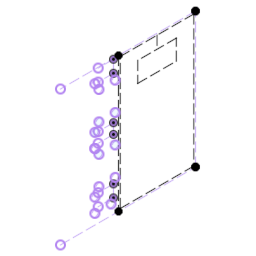
SAL v20 (Autodesk Fusion 360 design; units mm, degrees)
Autodesk Fusion 360 part; units mm, degrees
(part 1 of 3)
sketch "Sketch1" plane through (0, 0, 0) normal (0, 1, 0) x (1, 0, 0)
  line L0 (100, -100) -> (-100, -100) construction
  line L1 (-100, -100) -> (-100, 100) construction
  line L2 (-100, 100) -> (100, 100) construction
  line L3 (100, 100) -> (100, -100) construction
  line L4 (100, -100) -> (-100, 100) construction
  line L5 (-100, -100) -> (100, 100) construction
  line L6 (-105.5, -105.5) -> (-105.5, 105.5)
  line L7 (-105.5, 105.5) -> (105.5, 105.5)
  line L8 (105.5, 105.5) -> (105.5, -105.5)
  line L9 (105.5, -105.5) -> (-105.5, -105.5)
  line L10 (-95, -95) -> (-95, 95) construction
  line L11 (-95, 95) -> (95, 95) construction
  line L12 (95, 95) -> (95, -95) construction
  line L13 (95, -95) -> (-95, -95) construction
  line L14 (100, 100) -> (110, 100) construction
  line L15 (110, 100) -> (110, -100) construction
  line L16 (110, -100) -> (100, -100) construction
  line L17 (100, -100) -> (100, 100) construction
  line L18 (107.32, 100) -> (107.32, -100) construction
  line L19 (107.32, 90) -> (77.32, 90) construction
  line L20 (77.32, 90) -> (77.32, 10) construction
  line L21 (77.32, 10) -> (107.32, 10) construction
  line L22 (107.32, 10) -> (107.32, 90) construction
  line L23 (112.68, -100) -> (110, -100) construction
  line L24 (112.68, -100) -> (112.68, 100) construction
  line L25 (112.68, 100) -> (110, 100) construction
  line L26 (110, 0) -> (107.32, 0) construction
  line L27 (107.32, -100) -> (107.32, -105.5) construction
  line L28 (107.32, -105.5) -> (112.68, -105.5) construction
  line L29 (112.68, -105.5) -> (112.68, -100) construction
  line L30 (112.68, 100) -> (112.68, 105.5) construction
  line L31 (112.68, 105.5) -> (107.32, 105.5) construction
  line L32 (107.32, 105.5) -> (107.32, 100) construction
  line L33 (0, 0) -> (0, 110) construction
  line L34 (-100, 112.68) -> (100, 112.68)
  line L35 (100, 112.68) -> (100, 107.32)
  line L36 (100, 107.32) -> (-100, 107.32)
  line L37 (-100, 107.32) -> (-100, 112.68)
  line L38 (-100, 112.68) -> (100, 107.32) construction
  line L39 (100, 112.68) -> (-100, 107.32) construction
  line L40 (0, 0) -> (-105.5, 0) construction
  line L41 (100, -107.32) -> (-100, -107.32)
  line L42 (-88, -107.32) -> (-30, -107.32) construction
  line L43 (-30, -107.32) -> (-30, -42.32) construction
  line L44 (-30, -42.32) -> (-88, -42.32) construction
  line L45 (-88, -42.32) -> (-88, -107.32) construction
  line L46 (-107.32, 100) -> (-107.32, -100) construction
  line L47 (-112.68, -100) -> (-112.68, 100) construction
  point P0 (39.2, 88)
  point P1 (0, 110)
  dimension "d1" = 200
  dimension "d2" = -5.5
  dimension "d3" = 5
  dimension "d4" = 10
  dimension "d5" = 2.68
  dimension "d6" = 80
  dimension "d7" = 30
  dimension "d9" = 5
  dimension "d10" = 17.5
  dimension "d11" = 55.8
  dimension "d41" = 110
  dimension "d42" = 5.36
  dimension "d115" = 17.5
  dimension "d116" = 58
  dimension "d117" = 65
  constraint horizontal L0
  constraint perpendicular L0 L1
  constraint parallel L0 L2
  constraint parallel L1 L3
  constraint coincident L4 L33.start
  constraint coincident L5 L33.start
  constraint coincident L33.start L40.start
  constraint equal L2 L3
  constraint horizontal L14
  constraint vertical L15
  constraint horizontal L16
  constraint vertical L17
  constraint coincident L0.start L16
  constraint coincident L14 L18.start
  constraint coincident L16 L18.end
  constraint perpendicular L16 L18
  constraint horizontal L19
  constraint vertical L20
  constraint horizontal L21
  constraint vertical L22
  constraint coincident L18 L19.start
  constraint horizontal L23
  constraint perpendicular L23 L24
  constraint horizontal L25
  constraint midpoint L18 L26.end
  constraint midpoint L15 L26.start
  constraint equal L23 L26
  constraint perpendicular L16 L27
  constraint perpendicular L18 L28
  constraint coincident L23.start L24.start
  constraint vertical L29
  constraint coincident L8.end L28
  constraint perpendicular L25 L30
  constraint perpendicular L18 L31
  constraint perpendicular L14 L32
  constraint coincident L7.end L31
  constraint perpendicular L7 L33
  constraint horizontal L34
  constraint perpendicular L34 L35
  constraint parallel L34 L36
  constraint parallel L35 L37
  constraint coincident L38 P1
  constraint coincident L39 P1
  constraint coincident P1 L33.end
  constraint coincident L1.end L37
  constraint midpoint L6 L40.end
  constraint symmetric L35.end L40 L41.start
  constraint symmetric L36.end L40 L41.end
  constraint horizontal L42
  constraint vertical L43
  constraint horizontal L44
  constraint vertical L45
  constraint coincident L41 L42.start
  constraint symmetric L18.start L33 L46.start
  constraint symmetric L18.end L33 L46.end
  constraint symmetric L23.start L33 L47.start
  constraint symmetric L24.end L33 L47.end
  measures "d1" distance of L1.end L2.end
  measures "d4" distance of L15.end L0.start
  measures "d5" distance of L15 L18
  measures "d6" distance of L19.start L21.end
  measures "d7" distance of L20.end L21.end
  measures "d9" distance of L11.end L19
  measures "d10" distance of L7 P0
  measures "d11" distance of L12 P0
  measures "d41" distance of L33.start P1
  measures "d42" distance of L34.start L36.end
  measures "d115" distance of L6 L45
  measures "d116" distance of L42.start L42.end
  measures "d117" distance of L42.start L44.end
sketch "base_layer" plane through (0, 0, 0) normal (0, 1, 0) x (1, 0, 0)
  line L0 (-90, 90) -> (18, 90) construction
  line L1 (18, 90) -> (18, -10)
  line L2 (18, -10) -> (-90, -10) construction
  line L3 (-90, -10) -> (-90, 90) construction
  line L4 (-95, 95) -> (95, 95)
  line L5 (-68.2, 90) -> (-68.2, 39)
  line L6 (-68.2, 39) -> (-90, 39)
  line L7 (-87.5, -10) -> (-87.5, -6)
  line L8 (-82.5, -10) -> (-82.5, -6)
  arc A0 (-82.5, -6) -> (-87.5, -6) centre (-85, -6) ccw
  line L9 (-95, -95) -> (-95, 95)
  circle A1 centre (13, 87) radius 1.6
  circle A2 centre (-72.45, 43.25) radius 4.25
  line L10 (-90, 39) -> (-90, -10)
  line L11 (-87.5, -10) -> (-90, -10)
  line L12 (-82.5, -10) -> (18, -10)
  line L13 (-68.2, 90) -> (18, 90)
  circle A3 centre (22.25, 43.25) radius 4.25
  line L14 (-95, -95) -> (95, -95) construction
  line L15 (95, -95) -> (95, 95) construction
  line L16 (72.25, 90) -> (38.25, 90)
  line L17 (38.25, 90) -> (38.25, -6)
  line L18 (38.25, -6) -> (72.25, -6)
  line L19 (72.25, -6) -> (72.25, 90)
  line L20 (67.25, -6) -> (67.25, -1) construction
  line L21 (67.25, -1) -> (72.25, -1) construction
  line L22 (43.25, -6) -> (43.25, -1) construction
  line L23 (43.25, -1) -> (38.25, -1) construction
  line L24 (67.25, 90) -> (67.25, 85) construction
  line L25 (67.25, 85) -> (72.25, 85) construction
  line L26 (38.25, 85) -> (43.25, 85) construction
  line L27 (43.25, 85) -> (43.25, 90) construction
  line L28 (26.5, 43.25) -> (63.25, 43.25) construction
  line L29 (100, 100) -> (100, -100)
  line L30 (63.25, 90) -> (100, 90) construction
  point P0 (13, 87)
  point P1 (-63.2, 83.5)
  point P2 (-53.6, 83.5)
  point P3 (-44, 83.5)
  point P4 (-34.4, 83.5)
  point P5 (-24.8, 83.5)
  point P6 (5, 83.5)
  point P7 (63.25, 90)
  point P8 (67.25, -1)
  point P9 (43.25, -1)
  point P10 (43.25, 85)
  point P11 (67.25, 85)
  dimension "d12" = 100
  dimension "d13" = 108
  dimension "d14" = 5
  dimension "d15" = 51
  dimension "d16" = 21.8
  dimension "d17" = 3
  dimension "d18" = 5
  dimension "d19" = 2.5
  dimension "d20" = 5
  dimension "d21" = 4
  dimension "d22" = 5
  dimension "d23" = 3.2
  dimension "d28" = 9.6
  dimension "d29" = 0
  dimension "d30" = 5
  dimension "d31" = 13
  dimension "d38" = 8.5
  dimension "d39" = 6.5
  dimension "d52" = 5
  dimension "d54" = 34
  dimension "d55" = 96
  dimension "d56" = 9
  dimension "d57" = 5
  constraint horizontal L0
  constraint vertical L1
  constraint horizontal L2
  constraint vertical L3
  constraint coincident L0 L5.start
  constraint perpendicular L0 L5
  constraint coincident L3 L6.end
  constraint perpendicular L3 L6
  constraint coincident L2 L7.start
  constraint perpendicular L2 L7
  constraint coincident L2 L8.start
  constraint perpendicular L2 L8
  constraint horizontal L7.end L8.end
  constraint horizontal A0.centre L7.end
  constraint coincident L7.end A0.end
  constraint coincident P0 A1.centre
  constraint horizontal P5 P6
  constraint tangent L5 A2
  constraint tangent L6 A2
  constraint coincident L5.start L13.start
  constraint equal A2 A3
  constraint horizontal A2.centre A3.centre
  constraint tangent L1 A3
  constraint coincident L9.start L14.start
  constraint perpendicular L9 L14
  constraint coincident L4.end L15.end
  constraint vertical L15
  constraint horizontal L16
  constraint vertical L17
  constraint horizontal L18
  constraint vertical L19
  constraint coincident L16 P7
  constraint coincident L18 L20.start
  constraint perpendicular L18 L20
  constraint coincident L19 L21.end
  constraint perpendicular L19 L21
  constraint coincident L18 L22.start
  constraint perpendicular L18 L22
  constraint coincident L17 L23.end
  constraint perpendicular L17 L23
  constraint coincident L19 L25.end
  constraint perpendicular L19 L25
  constraint coincident L17 L26.start
  constraint perpendicular L17 L26
  constraint vertical L27
  constraint equal L26 L27
  constraint equal L24 L27
  constraint equal L24 L25
  constraint equal L23 L26
  constraint equal L22 L23
  constraint equal L20 L22
  constraint equal L20 L21
  constraint coincident P8 L20.end
  constraint coincident P9 L22.end
  constraint coincident P10 L26.end
  constraint coincident P11 L24.end
  constraint coincident A3 L28.start
  constraint perpendicular L17 L28
  constraint coincident A3.centre L28
  constraint vertical P7 L28.end
  constraint coincident L16 L27.end
  constraint coincident P7 L30.start
  constraint coincident L29 L30.end
  constraint perpendicular L29 L30
  constraint equal L28 L30
  constraint coincident L16 L24.start
  constraint vertical L24
  measures "d12" distance of L0.end L1.end
  measures "d13" distance of L0.start L0.end
  measures "d14" distance of L0 L4
  measures "d15" distance of L0 L6
  measures "d16" distance of L3 L5
  measures "d17" vertical distance of L0.end P0
  measures "d18" horizontal distance of L0.end P0
  measures "d19" distance of L2.end L7
  measures "d20" distance of L7 L8
  measures "d21" distance of L2 A0.centre
  measures "d22" distance of L3 L9
  measures "d23" diameter of A1
  measures "d30" distance of L5 P1
  measures "d31" distance of L1 P6
  measures "d38" diameter of A2
  measures "d39" distance of L0 P6
  measures "d52" distance of L4 L16
  measures "d54" distance of L16.start L16.end
  measures "d55" distance of L16.start L18.end
  measures "d56" distance of L16.start P7
  measures "d57" distance of L26.start P10
sketch "switch_screw_plan" plane through (0, 0, 0) normal (1, 0, 0) x (0, 0, -1)
  line L0 (0, 0) -> (0, 2.68) construction
  line L1 (0, 0) -> (0, -2.68) construction
  line L2 (0, 0) -> (10, 0) construction
  line L3 (10, 0) -> (10, 20) construction
  line L4 (10, 20) -> (0, 20) construction
  line L5 (0, 20) -> (0, 12) construction
  line L6 (0, 12) -> (0, 2.68)
  point P0 (0, 12)
  point P1 (0, 2.68)
  point P2 (0, 13.6)
  dimension "d32" = 5.36
  dimension "d33" = 10
  dimension "d34" = 20
  dimension "d35" = 8
  dimension "d36" = 9.32
  dimension "d37" = 1.6
  constraint coincident L0.start L1.start
  constraint vertical L0
  constraint parallel L0 L1
  constraint equal L0 L1
  constraint perpendicular L0 L2
  constraint perpendicular L2 L3
  constraint perpendicular L3 L4
  constraint coincident L0 L4.end
  constraint perpendicular L4 L5
  constraint coincident P0 L5.end
  constraint coincident P1 L0.end
  constraint coincident L5 P2
  measures "d32" distance of P1 L1.end
  measures "d33" distance of L0.start L2.end
  measures "d34" distance of L2.end L3.end
  measures "d35" distance of L4.end P0
  measures "d36" distance of P1 P0
  measures "d37" distance of P0 P2
sketch "back_board_0" plane through (0, 0, 0) normal (0, 0, 1) x (1, 0, 0)
  line L0 (0, 0) -> (0, 10) construction
  line L1 (0, 0) -> (0, -10) construction
  line L2 (0, 10) -> (0, 30) construction
  line L3 (0, 30) -> (0, 35.5) construction
  line L4 (100, 35.5) -> (-100, 35.5)
  line L5 (-100, 35.5) -> (-100, 4.5) construction
  line L6 (-100, 4.5) -> (100, 4.5)
  line L7 (100, 4.5) -> (100, 35.5) construction
  line L8 (100, 35.5) -> (-100, 4.5) construction
  line L9 (-100, 35.5) -> (100, 4.5) construction
  circle A0 centre (5, 20) radius 2.25
  circle A1 centre (-24.8, 20) radius 2.25
  circle A2 centre (-34.4, 20) radius 2.25
  circle A3 centre (-63.2, 20) radius 2.25
  circle A4 centre (-53.6, 20) radius 2.25
  circle A5 centre (-44, 20) radius 2.25
  line L10 (26.5, 0) -> (18, 0)
  line L11 (29.5, 4.5) -> (29.5, 35.5) construction
  line L12 (29.5, 20) -> (100, 20) construction
  line L13 (52.25, 20) -> (77.25, 20) construction
  circle A6 centre (52.25, 20) radius 1.1
  circle A7 centre (77.25, 20) radius 1.1
  line L14 (55.35, 14.2) -> (74.15, 14.2) construction
  line L15 (74.15, 14.2) -> (74.15, 25.8) construction
  line L16 (74.15, 25.8) -> (55.35, 25.8) construction
  line L17 (55.35, 25.8) -> (55.35, 14.2)
  line L18 (55.35, 14.2) -> (74.15, 25.8) construction
  line L19 (74.15, 14.2) -> (55.35, 25.8) construction
  arc A8 (74.15, 21.8) -> (70.15, 25.8) centre (70.15, 21.8) ccw
  arc A9 (70.15, 14.2) -> (74.15, 18.2) centre (70.15, 18.2) ccw
  line L20 (74.15, 18.2) -> (74.15, 21.8)
  line L21 (70.15, 25.8) -> (55.35, 25.8)
  line L22 (70.15, 14.2) -> (55.35, 14.2)
  line L23 (105.5, 0) -> (-105.5, 0)
  line L24 (-100, 4.5) -> (-105.5, 4.5)
  line L25 (-105.5, 4.5) -> (-105.5, 35.5)
  line L26 (-105.5, 35.5) -> (-100, 35.5)
  line L27 (100, 4.5) -> (105.5, 4.5)
  line L28 (105.5, 4.5) -> (105.5, 35.5)
  line L29 (105.5, 35.5) -> (100, 35.5)
  point P0 (0, 4.5)
  point P1 (0, 20)
  point P2 (100, 0)
  point P3 (0, 20)
  point P4 (5, 0)
  point P5 (-24.8, 0)
  point P6 (-34.4, 0)
  point P7 (-44, 0)
  point P8 (-53.6, 0)
  point P9 (-63.2, 0)
  point P10 (5, 20)
  point P11 (-24.8, 20)
  point P12 (-34.4, 20)
  point P13 (-44, 20)
  point P14 (-53.6, 20)
  point P15 (-63.2, 20)
  point P16 (64.75, 20)
  point P17 (52.25, 20)
  point P18 (77.25, 20)
  point P19 (64.75, 20)
  dimension "d43" = 20
  dimension "d44" = 20
  dimension "d45" = 5.5
  dimension "d46" = 5.5
  dimension "d47" = 4.5
  dimension "d51" = 3
  dimension "d104" = 25
  dimension "d105" = 2.2
  dimension "d106" = 18.8
  dimension "d107" = 11.6
  dimension "d108" = 4
  constraint coincident L0.start L1.start
  constraint vertical L0
  constraint parallel L0 L1
  constraint equal L0 L1
  constraint parallel L0 L2
  constraint coincident L0 P0
  constraint parallel L2 L3
  constraint midpoint L2 P3
  constraint horizontal L4
  constraint perpendicular L4 L5
  constraint parallel L4 L6
  constraint parallel L5 L7
  constraint coincident L8 P3
  constraint coincident L9 P3
  constraint coincident P3 P1
  constraint coincident P2 L7
  constraint coincident P0 L6
  constraint vertical P9 P15
  constraint vertical P8 P14
  constraint vertical P7 P13
  constraint vertical P6 P12
  constraint vertical P5 P11
  constraint vertical P4 P10
  constraint horizontal P3 P10
  constraint horizontal P3 P11
  constraint horizontal P3 P12
  constraint horizontal P3 P13
  constraint horizontal P3 P14
  constraint horizontal P3 P15
  constraint coincident P10 A0.centre
  constraint coincident P11 A1.centre
  constraint coincident P12 A2.centre
  constraint coincident P15 A3.centre
  constraint coincident P14 A4.centre
  constraint coincident P13 A5.centre
  constraint equal A0 A1
  constraint equal A1 A2
  constraint equal A1 A5
  constraint equal A1 A4
  constraint equal A1 A3
  constraint coincident L6 L11.start
  constraint coincident L4 L11.end
  constraint perpendicular L4 L11
  constraint midpoint L11 L12.start
  constraint midpoint L7 L12.end
  constraint midpoint L12 P19
  constraint coincident L12 P17
  constraint coincident L12 P18
  constraint coincident P17 L13.start
  constraint coincident P18 L13.end
  constraint parallel L12 L13
  constraint midpoint P19 L13
  constraint equal A6 A7
  constraint horizontal L14
  constraint perpendicular L14 L15
  constraint parallel L14 L16
  constraint parallel L15 L17
  constraint coincident L18 P19
  constraint coincident L19 P19
  constraint coincident P19 P16
  constraint horizontal A8.centre A8.start
  constraint vertical A8.centre A8.end
  constraint coincident L16 A8.end
  constraint coincident L15 A8.start
  constraint horizontal A9.centre A9.end
  constraint vertical A9.centre A9.start
  constraint equal A8 A9
  constraint coincident L15 A9.end
  constraint coincident L14 A9.start
  constraint coincident A9.end L20.start
  constraint perpendicular L5 L24
  constraint perpendicular L24 L25
  constraint horizontal L26
  constraint coincident L23.end L25
  constraint perpendicular L7 L27
  constraint perpendicular L27 L28
  constraint horizontal L29
  constraint coincident L23.start L28
  measures "d43" distance of L0.end L1.end
  measures "d44" distance of L0.end L2.end
  measures "d45" distance of L2.end L3.end
  measures "d46" distance of L0.end P0
  measures "d47" diameter of A0
  measures "d51" horizontal distance of L10.start L11.start
  measures "d104" distance of P17 P18
  measures "d105" diameter of A6
  measures "d106" distance of L15.end L16.end
  measures "d107" distance of L14.end L15.end
  measures "d108" radius of A8
sketch "left side panel" plane through (0, 0, 0) normal (1, 0, 0) x (0, 0, -1)
  line L0 (-120, 10) -> (120, 10) construction
  line L1 (120, 10) -> (120, -10) construction
  line L2 (120, -10) -> (-120, -10) construction
  line L3 (-120, -10) -> (-120, 10) construction
  line L4 (-120, 10) -> (120, -10) construction
  line L5 (120, 10) -> (-120, -10) construction
  line L6 (120, 10) -> (120, 230) construction
  line L7 (120, 230) -> (-120, 230) construction
  line L8 (-120, 230) -> (-120, 10) construction
  line L9 (-105.5, 215.5) -> (105.5, 215.5)
  line L10 (105.5, 215.5) -> (105.5, 4.5)
  line L11 (105.5, 4.5) -> (-105.5, 4.5)
  line L12 (-105.5, 4.5) -> (-105.5, 215.5)
  line L13 (-105.5, 215.5) -> (-120, 215.5) construction
  line L14 (-120, 215.5) -> (-120, 230) construction
  line L15 (-120, 230) -> (-105.5, 230) construction
  line L16 (-105.5, 230) -> (-105.5, 215.5) construction
  line L17 (-100, 10) -> (100, 10) construction
  line L18 (100, 10) -> (100, 210) construction
  line L19 (100, 210) -> (-100, 210) construction
  line L20 (-100, 210) -> (-100, 10) construction
  line L21 (100, 210) -> (105.5, 210) construction
  line L22 (105.5, 210) -> (105.5, 215.5) construction
  line L23 (105.5, 215.5) -> (100, 215.5) construction
  line L24 (100, 215.5) -> (100, 210) construction
  line L25 (10, 95) -> (90, 95) construction
  line L26 (90, 95) -> (90, 15) construction
  line L27 (90, 15) -> (10, 15) construction
  line L28 (10, 15) -> (10, 95) construction
  line L29 (10, 192.5) -> (90, 192.5) construction
  line L30 (90, 192.5) -> (90, 112.5) construction
  line L31 (90, 112.5) -> (10, 112.5) construction
  line L32 (10, 112.5) -> (10, 192.5) construction
  line L33 (90, 192.5) -> (90, 210) construction
  line L34 (90, 95) -> (90, 112.5) construction
  line L35 (10, 95) -> (14.25, 95) construction
  line L36 (14.25, 95) -> (14.25, 90.75) construction
  line L37 (14.25, 90.75) -> (10, 90.75) construction
  line L38 (10, 90.75) -> (10, 95) construction
  line L39 (90, 95) -> (85.75, 95) construction
  line L40 (85.75, 95) -> (85.75, 90.75) construction
  line L41 (85.75, 90.75) -> (90, 90.75) construction
  line L42 (90, 90.75) -> (90, 95) construction
  line L43 (10, 15) -> (14.25, 15) construction
  line L44 (14.25, 15) -> (14.25, 19.25) construction
  line L45 (14.25, 19.25) -> (10, 19.25) construction
  line L46 (10, 19.25) -> (10, 15) construction
  line L47 (90, 15) -> (85.75, 15) construction
  line L48 (85.75, 15) -> (85.75, 19.25) construction
  line L49 (85.75, 19.25) -> (90, 19.25) construction
  line L50 (90, 19.25) -> (90, 15) construction
  line L51 (90, 112.5) -> (85.75, 112.5) construction
  line L52 (85.75, 112.5) -> (85.75, 116.75) construction
  line L53 (85.75, 116.75) -> (90, 116.75) construction
  line L54 (90, 116.75) -> (90, 112.5) construction
  line L55 (90, 192.5) -> (85.75, 192.5) construction
  line L56 (85.75, 192.5) -> (85.75, 188.25) construction
  line L57 (85.75, 188.25) -> (90, 188.25) construction
  line L58 (90, 188.25) -> (90, 192.5) construction
  line L59 (10, 192.5) -> (14.25, 192.5) construction
  line L60 (14.25, 192.5) -> (14.25, 188.25) construction
  line L61 (14.25, 188.25) -> (10, 188.25) construction
  line L62 (10, 188.25) -> (10, 192.5) construction
  line L63 (10, 112.5) -> (14.25, 112.5) construction
  line L64 (14.25, 112.5) -> (14.25, 116.75) construction
  line L65 (14.25, 116.75) -> (10, 116.75) construction
  line L66 (10, 116.75) -> (10, 112.5) construction
  line L67 (90, 15) -> (90, 10) construction
  line L68 (14.25, 19.25) -> (85.75, 90.75) construction
  circle A0 centre (50, 55) radius 43.5 construction
  circle A1 centre (14.25, 90.75) radius 2.5
  circle A2 centre (85.75, 90.75) radius 2.5
  circle A3 centre (14.25, 19.25) radius 2.5
  circle A4 centre (85.75, 19.25) radius 2.5
  arc A5 (32.9047, 95) -> (10, 72.0953) centre (50, 55) ccw
  arc A6 (90, 72.0953) -> (67.0953, 95) centre (50, 55) ccw
  arc A7 (67.0953, 15) -> (90, 37.9047) centre (50, 55) ccw
  arc A8 (10, 37.9047) -> (32.9047, 15) centre (50, 55) ccw
  line L69 (10, 72.0953) -> (10, 37.9047)
  line L70 (32.9047, 15) -> (67.0953, 15)
  line L71 (90, 37.9047) -> (90, 72.0953)
  line L72 (67.0953, 95) -> (32.9047, 95)
  line L73 (90, 103.75) -> (10, 103.75) construction
  circle A9 centre (85.75, 116.75) radius 2.5
  circle A10 centre (14.25, 116.75) radius 2.5
  arc A11 (10, 135.4047) -> (32.9047, 112.5) centre (50, 152.5) ccw
  line L74 (67.0953, 112.5) -> (32.9047, 112.5)
  arc A12 (90, 169.5953) -> (67.0953, 192.5) centre (50, 152.5) ccw
  line L75 (32.9047, 192.5) -> (67.0953, 192.5)
  arc A13 (32.9047, 192.5) -> (10, 169.5953) centre (50, 152.5) ccw
  line L76 (10, 135.4047) -> (10, 169.5953)
  arc A14 (67.0953, 112.5) -> (90, 135.4047) centre (50, 152.5) ccw
  line L77 (90, 169.5953) -> (90, 135.4047)
  circle A15 centre (85.75, 188.25) radius 2.5
  circle A16 centre (14.25, 188.25) radius 2.5
  point P0 (0, 4.5)
  point P1 (0, 10)
  point P2 (90, 0)
  point P3 (85.75, 188.25)
  point P4 (14.25, 188.25)
  point P5 (14.25, 116.75)
  point P6 (85.75, 116.75)
  point P7 (85.75, 90.75)
  point P8 (14.25, 19.25)
  point P9 (14.25, 90.75)
  point P10 (85.75, 19.25)
  point P11 (90, 0)
  point P12 (50, 55)
  point P13 (-0.7942, 92.6847)
  dimension "d58" = 240
  dimension "d59" = 20
  dimension "d60" = 240
  dimension "d61" = 5.5
  dimension "d62" = 80
  dimension "d64" = 4.25
  dimension "d65" = 5
  dimension "d66" = 87
  dimension "d82" = 5
  constraint horizontal L0
  constraint perpendicular L0 L1
  constraint parallel L0 L2
  constraint parallel L1 L3
  constraint coincident L4 origin
  constraint coincident L5 origin
  constraint vertical L6
  constraint horizontal L7
  constraint vertical L8
  constraint coincident L0.end L1.start
  constraint horizontal L9
  constraint vertical L10
  constraint horizontal L11
  constraint vertical L12
  constraint midpoint L11 P0
  constraint vertical origin P0
  constraint equal L9 L10
  constraint horizontal L13
  constraint vertical L14
  constraint horizontal L15
  constraint vertical L16
  constraint equal L13 L16
  constraint horizontal L17
  constraint vertical L18
  constraint horizontal L19
  constraint vertical L20
  constraint coincident L0 L17.start
  constraint midpoint L17 P1
  constraint vertical P0 P1
  constraint equal L18 L19
  constraint horizontal L21
  constraint vertical L22
  constraint horizontal L23
  constraint vertical L24
  constraint equal L21 L24
  constraint horizontal L25
  constraint vertical L26
  constraint horizontal L27
  constraint vertical L28
  constraint equal L25 L28
  constraint horizontal L29
  constraint vertical L30
  constraint horizontal L31
  constraint vertical L32
  constraint equal L29 L30
  constraint collinear L26 L30
  constraint coincident L19 L33.end
  constraint perpendicular L19 L33
  constraint perpendicular L31 L34
  constraint equal L33 L34
  constraint horizontal L35
  constraint vertical L36
  constraint horizontal L37
  constraint vertical L38
  constraint horizontal L39
  constraint vertical L40
  constraint horizontal L41
  constraint vertical L42
  constraint horizontal L43
  constraint vertical L44
  constraint horizontal L45
  constraint vertical L46
  constraint horizontal L47
  constraint vertical L48
  constraint horizontal L49
  constraint vertical L50
  constraint horizontal L51
  constraint vertical L52
  constraint horizontal L53
  constraint vertical L54
  constraint horizontal L55
  constraint vertical L56
  constraint horizontal L57
  constraint vertical L58
  constraint horizontal L59
  constraint vertical L60
  constraint horizontal L61
  constraint vertical L62
  constraint horizontal L63
  constraint vertical L64
  constraint horizontal L65
  constraint vertical L66
  constraint equal L36 L37
  constraint equal L36 L64
  constraint equal L64 L65
  constraint equal L36 L40
  constraint equal L40 L41
  constraint equal L41 L49
  constraint equal L48 L49
  constraint equal L37 L45
  constraint equal L44 L45
  constraint equal L52 L64
  constraint equal L52 L53
  constraint equal L53 L57
  constraint equal L56 L57
  constraint equal L61 L65
  constraint equal L60 L61
  constraint coincident P3 L56.end
  constraint coincident P4 L60.end
  constraint coincident P5 L64.end
  constraint coincident P6 L52.end
  constraint coincident P7 L40.end
  constraint coincident P8 L44.end
  constraint coincident P9 L36.end
  constraint coincident P10 L48.end
  constraint coincident L0 L67.end
  constraint vertical L67
  constraint coincident L67 P11
  constraint midpoint L68 P12
  constraint coincident P12 A0.centre
  constraint equal A1 A2
  constraint equal A3 A4
  constraint equal A1 A3
  constraint coincident A0 A5.end
  constraint coincident L28 A5.end
  constraint coincident A0 A6.end
  constraint coincident L25 A6.end
  constraint coincident A0 A7.end
  constraint coincident L26 A7.end
  constraint coincident L28 A8.start
  constraint coincident L27 A8.end
  constraint coincident A0 A8.end
  constraint perpendicular L70 L71
  constraint perpendicular L71 L72
  constraint horizontal L70
  constraint midpoint L34 L73.start
  constraint perpendicular L34 L73
  constraint coincident L32 L73.end
  constraint symmetric A1 L73 A10
  constraint symmetric A2 L73 A9
  constraint symmetric A3 L73 A16
  constraint symmetric A4 L73 A15
  constraint symmetric A5.start L73 A11.end
  constraint symmetric A5.end L73 A11.start
  constraint symmetric A5 L73 A11
  constraint symmetric A6.start L73 A14.end
  constraint symmetric A6.end L73 L74.start
  constraint symmetric A6 L73 A14
  constraint symmetric A7.start L73 A12.end
  constraint symmetric A7.end L73 A12.start
  constraint symmetric A7 L73 A12
  constraint symmetric A8.start L73 A13.end
  constraint symmetric A8.end L73 L75.start
  constraint symmetric A8 L73 A13
  constraint equal L25 L29
  measures "d58" distance of L1.end L2.end
  measures "d59" distance of L0.end L1.end
  measures "d60" distance of L2.end L7.end
  measures "d61" distance of L0 L11
  measures "d62" distance of L25.start L25.end
  measures "d64" distance of P9 L37.end
  measures "d65" distance of L26.end L67.end
  measures "d66" diameter of A0
  measures "d82" diameter of A1
sketch "vertical_planning" plane through (0, 0, 0) normal (0, 0, 1) x (1, 0, 0)
  line L0 (100, 10) -> (-100, 10)
  line L1 (-100, 10) -> (-100, -10)
  line L2 (-100, -10) -> (100, -10)
  line L3 (100, -10) -> (100, 10)
  line L4 (100, 10) -> (-100, -10) construction
  line L5 (-100, 10) -> (100, -10) construction
  line L6 (100, 30) -> (-100, 30)
  line L7 (-100, 30) -> (-100, 10)
  line L8 (100, 10) -> (100, 30)
  line L9 (100, 50) -> (-100, 50)
  line L10 (-100, 50) -> (-100, 30)
  line L11 (100, 30) -> (100, 50)
  line L12 (100, 70) -> (-100, 70)
  line L13 (-100, 70) -> (-100, 50)
  line L14 (100, 50) -> (100, 70)
  line L15 (100, 90) -> (-100, 90)
  line L16 (-100, 90) -> (-100, 70)
  line L17 (100, 70) -> (100, 90)
  line L18 (100, 110) -> (-100, 110)
  line L19 (-100, 110) -> (-100, 90)
  line L20 (100, 90) -> (100, 110)
  line L21 (100, 130) -> (-100, 130)
  line L22 (-100, 130) -> (-100, 110)
  line L23 (100, 110) -> (100, 130)
  line L24 (100, 150) -> (-100, 150)
  line L25 (-100, 150) -> (-100, 130)
  line L26 (100, 130) -> (100, 150)
  line L27 (100, 170) -> (-100, 170)
  line L28 (-100, 170) -> (-100, 150)
  line L29 (100, 150) -> (100, 170)
  line L30 (100, 190) -> (-100, 190)
  line L31 (-100, 190) -> (-100, 170)
  line L32 (100, 170) -> (100, 190)
  line L33 (100, 210) -> (-100, 210)
  line L34 (-100, 210) -> (-100, 190)
  line L35 (100, 190) -> (100, 210)
  line L36 (100, 230) -> (-100, 230)
  line L37 (-100, 230) -> (-100, 210)
  line L38 (100, 210) -> (100, 230)
  line L39 (-100, 40) -> (100, 40) construction
  line L40 (-100, 80) -> (100, 80) construction
  line L41 (100, 120) -> (-100, 120) construction
  line L42 (-100, 160) -> (100, 160) construction
  line L43 (100, 200) -> (-100, 200) construction
  line L44 (100, 42.675) -> (-100, 42.675)
  line L45 (100, 37.325) -> (-100, 37.325)
  line L46 (-100, 82.675) -> (100, 82.675)
  line L47 (-100, 77.325) -> (100, 77.325)
  line L48 (100, 122.675) -> (-100, 122.675)
  line L49 (100, 162.675) -> (-100, 162.675)
  line L50 (100, 202.675) -> (-100, 202.675)
  line L51 (100, 197.325) -> (-100, 197.325)
  line L52 (100, 157.325) -> (-100, 157.325)
  line L53 (100, 117.325) -> (-100, 117.325)
  point P0 (-100, 0)
  point P1 (0, 10)
  dimension "d86" = 0
  dimension "d87" = 220
  dimension "d308" = 2.675
  dimension "d309" = 2.675
  dimension "d310" = 2.675
  dimension "d311" = 2.675
  dimension "d312" = 2.675
  constraint horizontal L0
  constraint perpendicular L0 L1
  constraint parallel L0 L2
  constraint parallel L1 L3
  constraint coincident L4 origin
  constraint coincident L5 origin
  constraint coincident P1 L0
  constraint coincident P0 L1
  constraint midpoint L10 L39.start
  constraint midpoint L11 L39.end
  constraint midpoint L16 L40.start
  constraint midpoint L17 L40.end
  constraint midpoint L23 L41.start
  constraint midpoint L22 L41.end
  constraint midpoint L28 L42.start
  constraint midpoint L29 L42.end
  constraint midpoint L35 L43.start
  constraint midpoint L34 L43.end
  constraint coincident L11 L44.start
  constraint coincident L10 L44.end
  constraint perpendicular L10 L44
  constraint symmetric L39 L44.start L45.start
  constraint symmetric L39 L44.end L45.end
  constraint coincident L16 L46.start
  constraint coincident L17 L46.end
  constraint perpendicular L17 L46
  constraint symmetric L40 L46.start L47.start
  constraint symmetric L40 L46.end L47.end
  constraint coincident L23 L48.start
  constraint coincident L22 L48.end
  constraint perpendicular L22 L48
  constraint coincident L29 L49.start
  constraint coincident L28 L49.end
  constraint perpendicular L28 L49
  constraint coincident L35 L50.start
  constraint coincident L34 L50.end
  constraint perpendicular L34 L50
  constraint symmetric L43 L50.start L51.start
  constraint symmetric L43 L50.end L51.end
  constraint symmetric L42 L49.start L52.start
  constraint symmetric L42 L49.end L52.end
  constraint symmetric L41 L48.start L53.start
  constraint symmetric L41 L48.end L53.end
  measures "d308" distance of L39 L44
  measures "d309" distance of L40 L46
  measures "d310" distance of L41 L48
  measures "d311" distance of L42 L49
  measures "d312" distance of L43 L50
extrude "Extrude1" add sketch "base_layer" along normal up to surface (1.6 mm away) from surface at 12 contours L1 L5 L6 L7 L8 A0 L10 L11 L12 L13 makes body 1
sketch "standoffs" plane through (0, 0, 0) normal (0, 1, 0) x (1, 0, 0)
  circle A0 centre (-72.45, 43.25) radius 4.25
  circle A1 centre (22.25, 43.25) radius 4.25
  circle A2 centre (-72.45, 43.25) radius 2.7
  circle A3 centre (-85, -6) radius 4.25
  circle A4 centre (22.25, 43.25) radius 2.7
  circle A5 centre (13, 87) radius 1.75
  circle A6 centre (13, 87) radius 4.25
  circle A7 centre (-85, -6) radius 2.7
  point P0 (-85, -6)
  point P1 (13, 87)
  dimension "d91" = 5.4
  dimension "d92" = 3.5
  constraint concentric A0 A2
  constraint coincident P0 A3.centre
  constraint concentric A1 A4
  constraint coincident P1 A5.centre
  constraint concentric A5 A6
  constraint equal A0 A3
  constraint equal A2 A4
  constraint equal A1 A6
  constraint equal A2 A7
  measures "d91" diameter of A2
  measures "d92" diameter of A5
extrude "Extrude2" add sketch "standoffs" along normal up to surface (9.12 mm away) from surface at 2.68 separate body contours A3 | A6 makes body 2 at (17.2447, 8.76, -86.7882) makes body 3 at (-80.7553, 8.76, 6.2118)
extrude "Extrude3" add sketch "standoffs" along normal blind 7 from surface at 2.68 separate body contours A0 | A1 makes body 4 at (26.4789, 7.3467, -42.8268) makes body 5 at (-68.2211, 7.3467, -42.8268)
sketch "bottom board laser cut" plane through (0, 0, 0) normal (0, 1, 0) x (1, 0, 0)
  line L0 (-105.5, -105.5) -> (-105.5, 105.5)
  line L1 (-105.5, 105.5) -> (105.5, 105.5)
  line L2 (105.5, 105.5) -> (105.5, -105.5)
  line L3 (105.5, -105.5) -> (-105.5, -105.5)
  line L4 (-90, -10) -> (-90, 90) construction
  line L5 (-90, 90) -> (18, 90) construction
  line L6 (95, -95) -> (95, 95) construction
  line L7 (-95, -95) -> (95, -95) construction
  circle A0 centre (-85, -6) radius 2
  circle A1 centre (-72.45, 43.25) radius 2
  circle A2 centre (22.25, 43.25) radius 2
  circle A3 centre (13, 87) radius 1.1
  circle A4 centre (43.25, -1) radius 0.9
  circle A5 centre (67.25, -1) radius 0.9
  circle A6 centre (67.25, 85) radius 0.9
  circle A7 centre (43.25, 85) radius 0.9
  line L8 (95, -95) -> (5, -95) construction
  line L9 (5, -95) -> (5, -80) construction
  line L10 (5, -80) -> (95, -80) construction
  line L11 (95, -80) -> (95, -95) construction
  circle A8 centre (5, -80) radius 0.9
  point P0 (-72.45, 43.25)
  point P1 (-85, -6)
  point P2 (22.25, 43.25)
  point P3 (13, 87)
  point P4 (43.25, -1)
  point P5 (67.25, -1)
  point P6 (67.25, 85)
  point P7 (43.25, 85)
  dimension "d99" = 4
  dimension "d100" = 2.2
  dimension "d101" = 1.8
  dimension "d102" = 90
  dimension "d103" = 15
  constraint coincident P1 A0.centre
  constraint coincident P0 A1.centre
  constraint coincident P2 A2.centre
  constraint coincident P3 A3.centre
  constraint coincident P4 A4.centre
  constraint coincident P5 A5.centre
  constraint coincident P6 A6.centre
  constraint coincident P7 A7.centre
  constraint equal A4 A5
  constraint equal A4 A7
  constraint equal A4 A6
  constraint equal A0 A1
  constraint equal A0 A2
  constraint horizontal L8
  constraint vertical L9
  constraint horizontal L10
  constraint vertical L11
  constraint coincident L6.start L7.end
  constraint coincident L9.end L10.start
  constraint equal A4 A8
  measures "d99" diameter of A0
  measures "d100" diameter of A3
  measures "d101" diameter of A4
  measures "d102" distance of L6.start L8.end
  measures "d103" distance of L6.start L10.end
sketch "amplifier_support" plane through (0, 0, 0) normal (0, 1, 0) x (1, 0, 0)
  line L0 (-2.5, -76.5) -> (12.5, -76.5) construction
  line L1 (12.5, -76.5) -> (12.5, -83.5)
  line L2 (12.5, -83.5) -> (-2.5, -83.5)
  line L3 (-2.5, -83.5) -> (-2.5, -76.5)
  line L4 (-2.5, -76.5) -> (12.5, -83.5) construction
  line L5 (12.5, -76.5) -> (-2.5, -83.5) construction
  line L6 (12.5, -76.5) -> (12.5, -74.5)
  line L7 (12.5, -74.5) -> (-2.5, -74.5)
  line L8 (-2.5, -74.5) -> (-2.5, -76.5)
  circle A0 centre (5, -80) radius 1.3
  point P0 (5, -80)
  point P1 (5, -80)
  dimension "d109" = 15
  dimension "d110" = 7
  dimension "d111" = 2
  dimension "d112" = 2.6
  constraint horizontal L0
  constraint perpendicular L0 L1
  constraint parallel L0 L2
  constraint parallel L1 L3
  constraint coincident L4 P1
  constraint coincident L5 P1
  constraint coincident P0 A0.centre
  constraint perpendicular L0 L6
  constraint perpendicular L6 L7
  constraint vertical L8
  constraint coincident P1 P0
  measures "d109" distance of L1.end L2.end
  measures "d110" distance of L0.end L1.end
  measures "d111" distance of L0.start L7.end
  measures "d112" diameter of A0
extrude "Extrude4" add sketch "amplifier_support" along normal blind 3 separate body makes body 6
sketch "Sketch10" plane through (0, 0, 0) normal (0, 0, 1) x (1, 0, 0)
  point P0 (100, 40)
  point P1 (100, 80)
  point P2 (100, 120)
  point P3 (100, 160)
  point P4 (100, 200)
  point P5 (77.32, 0)
sketch "intraboard_planning" plane through (0, 0, 0) normal (0, 1, 0) x (1, 0, 0)
  line L0 (-105.5, 105.5) -> (105.5, 105.5)
  line L1 (-30, -42.32) -> (-88, -42.32)
  line L2 (77.32, 90) -> (77.32, 10)
  line L3 (-100, -100) -> (-100, 100)
  line L4 (77.32, -41.5) -> (77.32, 10)
  line L5 (77.32, 90) -> (77.32, 105.5)
  line L6 (-84.68, -41.5) -> (-84.68, 105.5)
  line L7 (-107.32, 100) -> (-107.32, -100)
  line L8 (-84.68, -41.5) -> (77.32, -41.5)
  line L9 (-79.68, -41.5) -> (-79.68, -21.5)
  line L10 (-79.68, -21.5) -> (-84.68, -21.5)
  line L11 (-79.68, -41.5) -> (-79.68, -42.1)
  line L12 (-79.68, -42.1) -> (-85.28, -42.1)
  line L13 (-85.28, -42.1) -> (-85.28, -21.5)
  line L14 (-85.28, -21.5) -> (-84.68, -21.5)
  line L15 (-85.28, -21.5) -> (-107.32, -21.5)
  line L16 (-79.68, -42.1) -> (-79.68, -44.1)
  line L17 (-79.68, -44.1) -> (-107.32, -44.1)
  line L18 (107.32, 100) -> (107.32, -100)
  line L19 (72.32, -21.5) -> (77.32, -21.5)
  line L20 (77.32, -21.5) -> (77.92, -21.5)
  line L21 (77.92, -21.5) -> (77.92, -42.1)
  line L22 (77.92, -42.1) -> (72.32, -42.1)
  line L23 (72.32, -42.1) -> (72.32, -41.5)
  line L24 (72.32, -41.5) -> (72.32, -21.5)
  line L25 (72.32, -42.1) -> (72.32, -47.1)
  line L26 (72.32, -47.1) -> (107.32, -47.1)
  line L27 (77.92, -21.5) -> (107.32, -21.5)
  dimension "d119" = 22.64
  dimension "d120" = 0.82
  dimension "d122" = 5
  dimension "d123" = 20
  dimension "d126" = 0.6
  dimension "d127" = 2
  dimension "d130" = 5
  constraint coincident L2.end L4.end
  constraint vertical L4
  constraint coincident L2.start L5.start
  constraint coincident L0 L5.end
  constraint perpendicular L0 L5
  constraint coincident L0 L6.end
  constraint perpendicular L0 L6
  constraint horizontal L8
  constraint coincident L8 L9.start
  constraint perpendicular L8 L9
  constraint coincident L6 L10.end
  constraint perpendicular L6 L10
  constraint perpendicular L8 L11
  constraint perpendicular L11 L12
  constraint perpendicular L12 L13
  constraint horizontal L14
  constraint coincident L7 L15.end
  constraint perpendicular L7 L15
  constraint perpendicular L12 L16
  constraint coincident L7 L17.end
  constraint perpendicular L7 L17
  constraint coincident L4 L19.end
  constraint perpendicular L4 L19
  constraint perpendicular L4 L20
  constraint perpendicular L19 L21
  constraint perpendicular L21 L22
  constraint coincident L8 L23.end
  constraint perpendicular L8 L23
  constraint vertical L24
  constraint coincident L10 L19.start
  constraint equal L11 L14
  constraint equal L11 L23
  constraint equal L20 L23
  constraint equal L10 L19
  constraint perpendicular L22 L25
  constraint coincident L18 L26.end
  constraint perpendicular L18 L26
  constraint coincident L18 L27.end
  constraint perpendicular L18 L27
  constraint coincident L9.start L11.start
  measures "d119" distance of L6 L7
  measures "d120" distance of L1 L8
  measures "d122" distance of L9.end L10.end
  measures "d123" distance of L6.start L10.end
  measures "d126" distance of L9.start L11.end
  measures "d127" distance of L11.end L16.end
  measures "d130" distance of L22.end L25.end